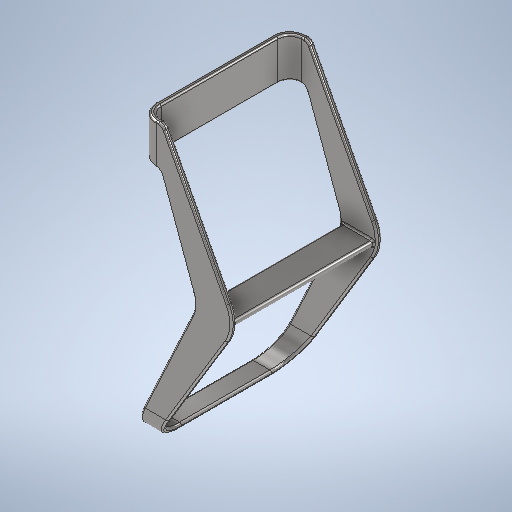
# Autodesk Inventor part: Chair 1
Saved by Autodesk Inventor 2025 (Build 290162000, 162)
## iProperties
Created: 2026-02-17
Part Number: Chair 1
Material: Steel, Alloy
Document SubType Name: Modeling
Designer: user
Density: 7.73 g/cm^3
Appearance: Semi-Polished
Author: user
Autodesk Inventor part; units mm, degrees
ref_plane "YZ Plane" through (0, 0, 0) normal (1, 0, 0) x (0, 1, 0)
ref_plane "XZ Plane" through (0, 0, 0) normal (0, 1, 0) x (-1, 0, 0)
ref_plane "XY Plane" through (0, 0, 0) normal (0, 0, 1) x (1, 0, 0)
sketch "Sketch1" plane through (0, 0, 0) normal (0, 0, 1) x (1, 0, 0)
  line L0 (0, 0) -> (60, 0)
  line L1 (60, 0) -> (320.5123, 430)
  line L2 (320.5123, 430) -> (100, 850)
  line L3 (100, 850) -> (30, 850)
  line L4 (30, 850) -> (30, 730)
  line L5 (30, 730) -> (91.3212, 730)
  line L6 (91.3212, 730) -> (200.5123, 430)
  line L7 (200.5123, 430) -> (0, 0)
  line L8 (70, 430) -> (470, 430)
  line L9 (470, 430) -> (585.2182, 0)
  point P0 (30, 790)
  dimension "d1" = 850
  dimension "d2" = 120
  dimension "d3" = 30
  dimension "d4" = 120
  dimension "d5" = 430
  dimension "d6" = 400
  dimension "d7" = 40
  dimension "d8" = 105
  dimension "d9" = 70
  dimension "d10" = 65
  dimension "d11" = 60
  dimension "d12" = 70
  constraints: 20 end point, 3 horizontal, 3 horizontal alignment, 2 perpendicular, 1 midpoint
  measures "d1" distance from line of L0.start L3
  measures "d2" distance of L3.end L4.end
  measures "d3" horizontal distance of L0.start point (30, 790)
  measures "d4" distance of L1.end L6.end
  measures "d5" vertical distance of L0.start L1.end
  measures "d6" distance of L8.start L8.end
  measures "d7" horizontal distance of L8.start L4.end
  measures "d8" angle of L9 L8
  measures "d9" angle of L8 L6
  measures "d10" angle of L7 L8
  measures "d11" distance of L0.start L0.end
  measures "d12" distance of L2.end L3.end
extrude "Extrusion1" add sketch "Sketch1" along normal mid plane 450
fillet "Fillet1" radius 20 2 edges at (100, 850, 0) (91.3212, 730, 0)
fillet "Fillet2" radius 90 2 edges at (30, 0, 225) (30, 0, -225)
fillet "Fillet3" radius 80 1 edges at (200.5123, 430, 0)
fillet "Fillet4" radius 100 1 edges at (320.5123, 430, 0)
fillet "Fillet5" radius 50 2 edges at (30, 790, 225) (30, 790, -225)
shell "Shell1" thickness 15 removed faces 10 at (296.1699, 476.1666, 75) at (104.8995, 840.5552, 75) at (232.3417, 284.4661, 75) at (68.6077, 850, -58.3333) at (231.38, 599.7664, 75) at (193.2248, 444.9109, -75) at (158.1561, 546.3726, 75) at (95.5662, 718.1834, -75) at (61.5447, 730, 58.3333) at (90.1478, 193.3225, 75)
fillet "Fillet6" radius 5 64 edges at (98.2571, 847.1164, 210) (83.9558, 850, 210) (55.2513, 850, 199.7487) (45, 850, 0) (55.2513, 850, -199.7487) (83.9558, 850, -210) (98.2571, 847.1164, -210) (199.9398, 659.6491, -210) (305.6747, 430.4544, -210) (202.8877, 235.8496, -210) (82.3962, 36.967, -188.033) (69.0876, 15, 0) (82.3962, 36.967, 188.033) (202.8877, 235.8496, 210) (305.6747, 430.4544, 210) (199.9398, 659.6491, 210) (98.2571, 847.1164, 225) (83.9558, 850, 225) (44.6447, 850, 210.3553) (30, 850, 0) (44.6447, 850, -210.3553) (83.9558, 850, -225) (98.2571, 847.1164, -225) (199.9398, 659.6491, -225) (305.6747, 430.4544, -225) (202.8877, 235.8496, -225) (75.9702, 26.3604, -198.6396) (60, 0, 0) (75.9702, 26.3604, 198.6396) (202.8877, 235.8496, 225) (305.6747, 430.4544, 225) (199.9398, 659.6491, 225) (12.2921, 26.3604, 198.6396) (0, 0, 0) (12.2921, 26.3604, -198.6396) (114.2378, 244.9838, -225) (193.9272, 430.2875, -225) (142.6448, 588.9895, -225) (89.864, 725.5748, -225) (78.6636, 729.9546, -224.9821) (43.7085, 730, -209.3937) (30, 730, 0) (43.7085, 730, 209.3937) (78.6636, 729.9546, 224.9821) (89.864, 725.5748, 225) (142.6448, 588.9895, 225) (193.9272, 430.2875, 225) (114.2378, 244.9838, 225) (193.9272, 430.2875, -210) (142.6448, 588.9895, -210) (89.864, 725.5748, -210) (78.6631, 729.9547, -209.9745) (54.3202, 730, -198.7813) (45, 730, 0) (54.3202, 730, 198.7813) (78.6626, 729.9547, 209.9744) (89.864, 725.5748, 210) (142.6448, 588.9895, 210) (193.9272, 430.2875, 210) (114.2378, 244.9838, 210) (17.238, 36.967, 188.033) (6.9946, 15, 0) (17.238, 36.967, -188.033) (114.2378, 244.9838, -210)
sketch "Sketch2" plane through (47.4846, 90, -210) normal (0, 0, 1) x (1, 0, 0)
  arc A0 (139.0234, 309.9676) -> (141.6942, 371.1387) centre (66.5188, 343.7771) ccw construction
  arc A1 (243.765, 291.6991) -> (246.7757, 390.0011) centre (158.237, 343.5157) ccw construction
  line L0 (108.2432, 275.5197) -> (232.7468, 276.8203) construction
  line L1 (162.3163, 332.871) -> (242.3163, 332.871) construction
  line L2 (162.3163, 325.371) -> (242.3163, 325.371)
  line L3 (242.3163, 340.371) -> (162.3163, 340.371)
  arc A2 (162.3163, 340.371) -> (162.3163, 325.371) centre (162.3163, 332.871) ccw
  arc A3 (242.3163, 325.371) -> (242.3163, 340.371) centre (242.3163, 332.871) ccw
  arc A4 (139.0234, 309.9676) -> (141.6942, 371.1387) centre (66.5188, 343.7771) ccw construction
  arc A5 (243.765, 291.6991) -> (246.7757, 390.0011) centre (158.237, 343.5157) ccw construction
  arc A6 (139.0234, 309.9676) -> (141.6942, 371.1387) centre (66.5188, 343.7771) ccw construction
  line L4 (146.4426, 340.2875) -> (258.1901, 340.4544) construction
  point P0 (-47.4846, -90)
  point P1 (202.3163, 332.871)
  point P2 (202.3163, 340.371)
  dimension "d22" = 7.5
  dimension "d23" = 80
  constraints: 12 end point, 9 point on circle, 4 tangent, 2 centre point, 2 midpoint, 1 horizontal, 1 horizontal alignment, 1 parallel, 1 vertical alignment
  measures "d22" radius of A3
  measures "d23" distance of L1.start L1.end
extrude "Extrusion2" add sketch "Sketch2" along normal up to surface (420 mm away)
fillet "Fillet7" radius 5 8 edges at (297.3009, 422.871, -210) (249.8009, 415.371, -210) (202.3009, 422.871, -210) (249.8009, 430.371, -210) (202.3009, 422.871, 210) (249.8009, 415.371, 210) (297.3009, 422.871, 210) (249.8009, 430.371, 210)
body "Solid1"
